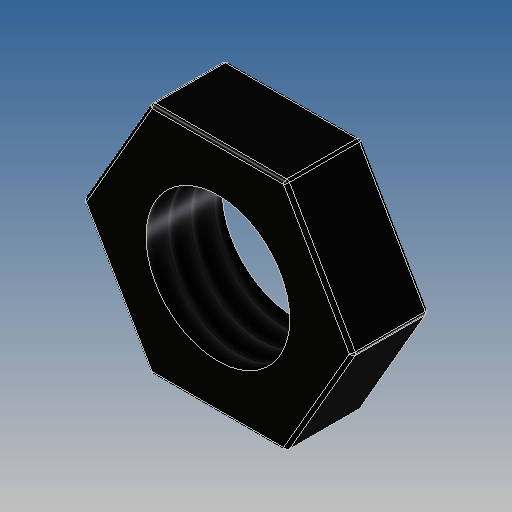
# Autodesk Inventor part: Large Nut
Saved by Autodesk Inventor 2018 (Build 220112000, 112)
## iProperties
Created: 2018-04-08
Part Number: Large Nut
Material: Stainless Steel
Document SubType Name: Modeling
Designer: Cole
Density: 8 g/cm^3
Appearance: Semi-Polished
Mass: 18.9475 g
Surface Area: 15.5937 cm^2
Volume: 2.36844 cm^3
Author: Cole
Autodesk Inventor part; units mm, degrees
ref_plane "YZ Plane" through (0, 0, 0) normal (1, 0, 0) x (0, 1, 0)
ref_plane "XZ Plane" through (0, 0, 0) normal (0, 1, 0) x (-1, 0, 0)
ref_plane "XY Plane" through (0, 0, 0) normal (0, 0, 1) x (1, 0, 0)
sketch "Sketch1" plane through (0, 0, 0) normal (0, 0, 1) x (1, 0, 0)
  line L0 (13.4938, 0) -> (6.7469, -11.6859)
  line L1 (6.7469, -11.6859) -> (-6.7469, -11.6859)
  line L2 (-6.7469, -11.6859) -> (-13.4938, 0)
  line L3 (-13.4938, 0) -> (-6.7469, 11.6859)
  line L4 (-6.7469, 11.6859) -> (6.7469, 11.6859)
  line L5 (6.7469, 11.6859) -> (13.4938, 0)
  circle A0 centre (0, 0) radius 7.1755
  point P0 (0, 0)
  point P1 (0, 0)
  dimension "d0" = 26.9875
  dimension "d1" = 14.351
  constraints: 12 end point, 1 centre point, 1 coincident, 13 other
  measures "d0" distance of L0.start L2.end
  measures "d1" diameter of A0
extrude "Extrusion1" add sketch "Sketch1" along normal blind 7.62
fillet "Fillet1" radius 0.3175 18 edges at (0, 11.6859, 7.62) (6.7469, 11.6859, 3.81) (-6.7469, 11.6859, 3.81) (0, 11.6859, 0) (10.1203, 5.843, 7.62) (10.1203, 5.843, 0) (13.4938, 0, 3.81) (10.1203, -5.843, 0) (10.1203, -5.843, 7.62) (6.7469, -11.6859, 3.81) (0, -11.6859, 7.62) (0, -11.6859, 0) (-6.7469, -11.6859, 3.81) (-10.1203, -5.843, 0) (-10.1203, -5.843, 7.62) (-13.4938, 0, 3.81) (-10.1203, 5.843, 7.62) (-10.1203, 5.843, 0)
thread "Thread1" size "5/8-11 UNC" class "2B" standard "ANSI Unified Screw Threads" full length
body "Solid1"
